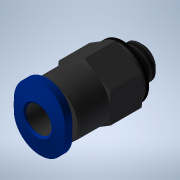
# Autodesk Inventor part: 153304 QSM-M5-4
Saved by Autodesk Inventor 2021 (Build 250183000, 183)
## iProperties
Created: 2026-04-07
Part Number: 153304 QSM-M5-4
Material: Generic
Catalog Web Link: www.3dfindit.com
Description: QSM-push-in fitting
Vendor: FESTO
Document SubType Name: Modeling
Designer: psAdmin
Manufacturer: FESTO
Mass: 3.2 g
Surface Area: 7.28863 cm^2
Volume: 0.570299 cm^3
Density: 1 g/cm^3
Appearance: PSOLRGB-176-176-176
Category: PARTsolutions
Company: FESTO
Title: 153304 QSM-M5-4
Author: Cadenas PARTsolutions
Comments: push-in fitting
PSOL_IDENT_0: {$CADENAS_DATA/23d-libs/festo/parts/q/qsm/qsm.prj},167 {VTYP=3D},{NB=153304 QSM-M5-4},{LINA=153304 Q
PSOL_IDENT_1: SM-M5-4},{NN=QSM},{DATE=02.05.2025 12:41:56},{GEOMDATE=01.04.2025 10:00:41},{VERSION=},{LINEID=40},{
PSOL_IDENT_2: WBVAR=},{WBNUMERIC=}  {NB=153304 QSM-M5-4},{LINA=153304 QSM-M5-4},{KT=1},{TNR=153304},{TYP=QSM-M5-4}
PSOL_IDENT_3: ,{TYPE=1.000},{FDT=1},{FDTQS=46},{FDTQS1=34},{FDTQS2=46},{FDTQSDZX=46},{ZOLL=5},{ZOLLDRVS=5},{ZOLLDF
PSOL_IDENT_4: M=5},{ZOLLDFMCN=5},{ZOLLAXNS=5},{ZOLLDZX=5},{D=M5},{D1=4},{BR=0.000},{A=3.000},{B=16.200},{C=11.500}
PSOL_IDENT_5: ,{L=13.200},{T=-},{X=7.800},{Y=9.800},{Z=0.000},{DD=0.000},{NENN=2.200},{DN=5.000},{DK=4.019},{BZE=0
PSOL_IDENT_6: .000},{D2=8.000},{L1=3.500},{L2=0.000},{SW=8.000},{D3=3.500},{I=0.000},{A1=0.000},{L5=0.000},{HEX=0.
PSOL_IDENT_7: 000},{P=0.000},{MOM=1.33 ±0.27},{CNSMASSEXACT=0.00320},{LSW=5.076923},{GTIN=4052568033699},{REACH=Ja
PSOL_IDENT_8: },{REACHSVHC=Ja},{REACHHAZSUBS=7439-92-1},{REACHSCIP=3732228b-b396-49b9-8f0d-ee75d35d3f40},{REACHVAL
PSOL_IDENT_9: DATE=05.03.2025}
NB: 153304 QSM-M5-4
NN: QSM
NT: push-in fitting
NBSYN: $TNR. $TYP.
LINA: 153304 QSM-M5-4
CATALOG: Festo
TNR: 153304
TYP: QSM-M5-4
D: M5
D1: 4
A: 3
B: 16.2
C: 11.5
L: 13.2
T: -
X: 7.8
Y: 9.8
Z: 0
NENN: 2.2
D2: 8
L1: 3.5
L2: 0
SW: 8
A1: 0
L5: 0
HEX: 0
P: 0
MOM: 1.33 ±0.27
CNSMASSEXACT: 0.0032
GTIN: 4052568033699
REACH: Yes
REACHSVHC: Yes
REACHHAZSUBS: 7439-92-1
REACHVALDATE: 05.03.2025
SUPPLIER: FESTO
ARTICLENO: 153304 QSM-M5-4
BOMINFO: 153304 QSM-M5-4
CREATOR: CADENAS GmbH
Autodesk Inventor part; units mm, degrees
sketch "Sketch_13" plane through (0, 0, 0) normal (1, 0, 0) x (0, 1, 0)
  line L0 (0, 0) -> (0, 13.2)
  line L1 (0, 13.2) -> (2.3, 13.2)
  line L2 (2.3, 13.2) -> (4.9347, 12.7354)
  arc A0 (5.1, 12.5385) -> (4.9347, 12.7354) centre (4.9, 12.5385) ccw
  line L3 (5.1, 12.5385) -> (5.1, 11.7)
  line L4 (5.1, 11.7) -> (3.075, 11.7)
  arc A1 (3.075, 11.7) -> (2.7, 11.325) centre (3.075, 11.325) ccw
  line L5 (2.7, 11.325) -> (2.7, 10.9)
  line L6 (2.7, 10.9) -> (3.9, 10.9)
  line L7 (3.9, 10.9) -> (3.9, 10.6)
  line L8 (3.9, 10.6) -> (3.9476, 10.6)
  line L9 (3.9476, 10.6) -> (4, 9.6)
  line L10 (4, 9.6) -> (4, 6.0769)
  line L11 (4, 6.0769) -> (4.64, 5.9054)
  line L12 (4.64, 5.9054) -> (4.64, 1.1715)
  line L13 (4.64, 1.1715) -> (4, 1)
  line L14 (4, 1) -> (4, 0.55)
  line L15 (4, 0.55) -> (3.95, 0.5)
  line L16 (3.95, 0.5) -> (4, 0.45)
  line L17 (4, 0.45) -> (4, 0)
  line L18 (4, 0) -> (0, 0)
  line L19 (0, 0) -> (0, 13.2)
  constraints: 40 end point, 4 point on circle, 2 centre point
revolve "Revolution1" add sketch "Sketch_13" angle 360 about axis through (0, 0, 0) along (0, 0, 1)
sketch "Sketch_14" plane through (0, 0, 13.2) normal (0, 0, 1) x (1, 0, 0)
  line L0 (-5.88, -3.3948) -> (0, -6.7896)
  line L1 (0, -6.7896) -> (5.88, -3.3948)
  line L2 (5.88, -3.3948) -> (5.88, 3.3948)
  line L3 (5.88, 3.3948) -> (0, 6.7896)
  line L4 (0, 6.7896) -> (-5.88, 3.3948)
  line L5 (-5.88, 3.3948) -> (-5.88, -3.3948)
  line L6 (-3.9, 1) -> (-3.9, -1)
  arc A0 (-3.9, -1) -> (0, -4.9) centre (0, -1) ccw
  arc A1 (0, -4.9) -> (3.9, -1) centre (0, -1) ccw
  line L7 (3.9, -1) -> (3.9, 1)
  arc A2 (3.9, 1) -> (0, 4.9) centre (0, 1) ccw
  arc A3 (0, 4.9) -> (-3.9, 1) centre (0, 1) ccw
  constraints: 16 end point, 8 point on circle, 4 centre point
extrude "Extrusion1" cut sketch "Sketch_14" against normal blind 1.5
sketch "Sketch_1" plane through (0, 0, 0) normal (0, 0, 1) x (1, 0, 0)
  line L0 (-8, -8) -> (8, -8)
  line L1 (8, -8) -> (8, 8)
  line L2 (8, 8) -> (-8, 8)
  line L3 (-8, 8) -> (-8, -8)
  line L4 (-4, -2.3094) -> (0, -4.6188)
  line L5 (0, -4.6188) -> (4, -2.3094)
  line L6 (4, -2.3094) -> (4, 2.3094)
  line L7 (4, 2.3094) -> (0, 4.6188)
  line L8 (0, 4.6188) -> (-4, 2.3094)
  line L9 (-4, 2.3094) -> (-4, -2.3094)
  constraints: 20 end point
extrude "Extrusion2" cut sketch "Sketch_1" along normal blind 7.7
sketch "Sketch_2" plane through (0, 0, 0) normal (1, 0, 0) x (0, 1, 0)
  line L0 (0, -3) -> (0, 0)
  line L1 (0, 0) -> (2.5, 0)
  line L2 (2.5, 0) -> (2.5, -2.5095)
  line L3 (2.5, -2.5095) -> (2.0095, -3)
  line L4 (2.0095, -3) -> (0, -3)
  line L5 (0, -3) -> (0, 0)
  constraints: 12 end point
revolve "Revolution2" add sketch "Sketch_2" angle 360 about axis through (0, 0, -3) along (0, 0, -1)
thread "Thread1" size "M5x0.8" class "6g" standard "ISO Metric profile" full length
sketch "Sketch_11" plane through (0, 0, 0) normal (1, 0, 0) x (0, 1, 0)
  line L0 (0, -3) -> (0, 13.2)
  line L1 (0, 13.2) -> (2.3, 13.2)
  arc A0 (2.3, 13.2) -> (2, 12.9) centre (2.3, 12.9) ccw
  line L2 (2, 12.9) -> (2, 1.7)
  line L3 (2, 1.7) -> (1.1, 1.7)
  line L4 (1.1, 1.7) -> (1.1, -3)
  line L5 (1.1, -3) -> (0, -3)
  line L6 (0, -3) -> (0, 13.2)
  constraints: 14 end point, 2 point on circle, 1 centre point
revolve "Revolution3" cut sketch "Sketch_11" angle 360 about axis through (0, 0, -3) along (0, 0, 1)
ref_plane "ANBAU_XY" through (0, 0, 0) normal (0, 0, -1) x (1, 0, 0)
ref_plane "ANBAU_YZ" through (0, 0, 0) normal (1, 0, 0) x (0, -1, 0)
ref_plane "ANBAU_ZX" through (0, 0, 0) normal (0, -1, 0) x (0, 0, -1)
ref_plane "ANBAU_STD_XY" through (0, 0, 0) normal (0, 0, 1) x (1, 0, 0)
ref_plane "ANBAU_STD_YZ" through (0, 0, 0) normal (1, 0, 0) x (0, 1, 0)
ref_plane "ANBAU_STD_ZX" through (0, 0, 0) normal (0, 1, 0) x (0, 0, 1)
ref_plane "FDT_ANBAU_XY" through (0, 0, 0) normal (0, 0, -1) x (1, 0, 0)
ref_plane "FDT_ANBAU_YZ" through (0, 0, 0) normal (1, 0, 0) x (0, -1, 0)
ref_plane "FDT_ANBAU_ZX" through (0, 0, 0) normal (0, -1, 0) x (0, 0, -1)
ref_plane "FDT_SCHLAUCH_XY" through (0, 0, 1.7) normal (0, 0, 1) x (1, 0, 0)
ref_plane "FDT_SCHLAUCH_YZ" through (0, 0, 1.7) normal (1, 0, 0) x (0, 1, 0)
ref_plane "FDT_SCHLAUCH_ZX" through (0, 0, 1.7) normal (0, 1, 0) x (0, 0, 1)
body "Solid1"
